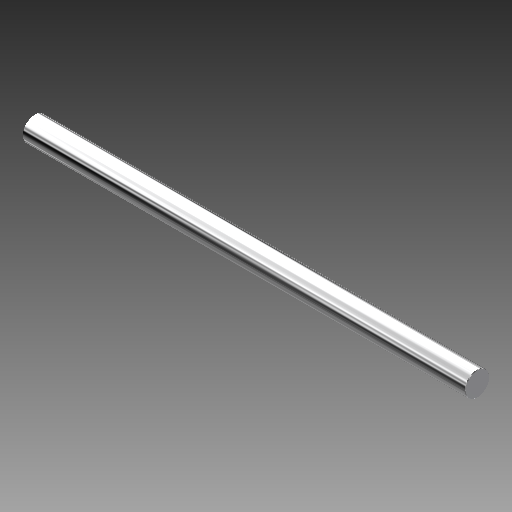
# Autodesk Inventor part: Eje Principal - Interno
Saved by Autodesk Inventor 2019 (Build 230136000, 136)
## iProperties
Created: 2019-09-30
Part Number: Eje Principal - Interno
Material: Aluminum 6061
Document SubType Name: Modeling
Designer: Domenico
Density: 2.7 g/cm^3
Appearance: Aluminum - Flat
CustomPartVersion: 1
Author: Domenico
Autodesk Inventor part; units mm, degrees
ref_plane "Start Plane" through (0, 0, 0) normal (1, 0, 0) x (0, 1, 0)
ref_plane "XZ Plane" through (0, 0, 0) normal (0, 1, 0) x (-1, 0, 0)
ref_plane "XY Plane" through (0, 0, 0) normal (0, 0, 1) x (1, 0, 0)
sketch "Main Sketch" plane through (0, 0, 0) normal (0, 0, 1) x (1, 0, 0)
  line L0 (0, 0) -> (460, 0)
  line L1 (460, 12.7) -> (460, 0)
  line L2 (10, 12.7) -> (460, 12.7)
  line L3 (0, 0) -> (0, 12.7)
  line L4 (0, 12.7) -> (10, 12.7)
  dimension "d3" = 25.4
  dimension "d15" = 25.4
  constraints: 10 end point, 2 horizontal, 2 vertical
  measures "d3" diameter of L2 L0
  measures "d15" diameter of L4 L0
revolve "Revolution1" add sketch "Main Sketch" angle 360 about axis through (0, 0, 0) along (1, 0, 0)
chamfer "Chamfer4" distance 0.595 angle 45 1 edges at (0, -12.7, 0) measured on face at (0.5, -12.7, 0)
chamfer "Chamfer3" distance 0.595 angle 45 1 edges at (460, -12.7, 0) measured on face at (459.5, -12.7, 0)
body "Solid1"
